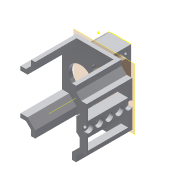
# Autodesk Inventor part: 30_Cube_Z_Focus_MGN_NEMA_base_v3
Saved by Autodesk Inventor 2019.4 (Build 234330000, 330)
## iProperties
Created: 2021-04-25
Part Number: 30_Cube_Z_Focus_MGN_NEMA_base_v3
Material: Generic
Document SubType Name: Modeling
Designer: diederichbenedict
Density: 1 g/cm^3
Appearance: Smooth - White
Author: diederichbenedict
Autodesk Inventor part; units mm, degrees
ref_plane "YZ Plane" through (0, 0, 0) normal (1, 0, 0) x (0, 1, 0)
ref_plane "XZ Plane" through (0, 0, 0) normal (0, 1, 0) x (-1, 0, 0)
ref_plane "XY Plane" through (0, 0, 0) normal (0, 0, 1) x (1, 0, 0)
ref_plane "Work Plane1" through (0, 0, 0) normal (0, 0, 1) x (1, 0, 0)
sketch "Sketch1" plane through (0, 0, 0) normal (0, 0, 1) x (1, 0, 0)
  arc A0 (24.85, 22.85) -> (22.85, 24.85) centre (22.85, 22.85) ccw construction
  line L0 (22.85, 24.85) -> (-16.97, 24.85) construction
  line L1 (-16.97, 24.85) -> (-16.97, 21.15) construction
  line L2 (-16.97, 21.15) -> (16.97, 21.15) construction
  line L3 (16.97, 16.97) -> (16.97, 21.15) construction
  line L4 (21.15, 16.97) -> (16.97, 16.97) construction
  line L5 (21.15, 16.97) -> (21.15, -16.97) construction
  line L6 (21.15, -16.97) -> (24.85, -16.97) construction
  line L7 (24.85, -16.97) -> (24.85, 22.85) construction
  line L8 (23.75, 23.25) -> (23.75, 18.15) construction
  arc A1 (23.25, 17.65) -> (23.75, 18.15) centre (23.25, 18.15) ccw construction
  line L9 (23.25, 17.65) -> (20.8937, 17.65) construction
  arc A2 (20.5239, 17.8134) -> (20.8937, 17.65) centre (20.8937, 18.15) ccw construction
  line L10 (20.5239, 17.8134) -> (17.7803, 20.8273) construction
  arc A3 (17.65, 21.1639) -> (17.7803, 20.8273) centre (18.15, 21.1639) ccw construction
  line L11 (17.65, 21.1639) -> (17.65, 23.25) construction
  arc A4 (18.15, 23.75) -> (17.65, 23.25) centre (18.15, 23.25) ccw construction
  line L12 (18.15, 23.75) -> (23.25, 23.75) construction
  arc A5 (23.75, 23.25) -> (23.25, 23.75) centre (23.25, 23.25) ccw construction
  arc A6 (-24.85, -22.85) -> (-22.85, -24.85) centre (-22.85, -22.85) ccw construction
  line L13 (-22.85, -24.85) -> (16.97, -24.85) construction
  line L14 (16.97, -24.85) -> (16.97, -21.15) construction
  line L15 (16.97, -21.15) -> (-16.97, -21.15) construction
  line L16 (-16.97, -16.97) -> (-16.97, -21.15) construction
  line L17 (-21.15, -16.97) -> (-16.97, -16.97) construction
  line L18 (-21.15, -16.97) -> (-21.15, 16.97) construction
  line L19 (-21.15, 16.97) -> (-24.85, 16.97) construction
  line L20 (-24.85, 16.97) -> (-24.85, -22.85) construction
  line L21 (-20.8273, -17.7803) -> (-17.8134, -20.5239) construction
  arc A7 (-17.65, -20.8937) -> (-17.8134, -20.5239) centre (-18.15, -20.8937) ccw construction
  line L22 (-17.65, -20.8937) -> (-17.65, -23.25) construction
  arc A8 (-18.15, -23.75) -> (-17.65, -23.25) centre (-18.15, -23.25) ccw construction
  line L23 (-18.15, -23.75) -> (-23.25, -23.75) construction
  arc A9 (-23.75, -23.25) -> (-23.25, -23.75) centre (-23.25, -23.25) ccw construction
  line L24 (-23.75, -23.25) -> (-23.75, -18.15) construction
  arc A10 (-23.25, -17.65) -> (-23.75, -18.15) centre (-23.25, -18.15) ccw construction
  line L25 (-23.25, -17.65) -> (-21.1639, -17.65) construction
  arc A11 (-20.8273, -17.7803) -> (-21.1639, -17.65) centre (-21.1639, -18.15) ccw construction
  arc A12 (-22.85, 24.85) -> (-24.85, 22.85) centre (-22.85, 22.85) ccw construction
  line L26 (-22.85, 24.85) -> (16.97, 24.85) construction
  line L27 (16.97, 24.85) -> (16.97, 21.15) construction
  line L28 (16.97, 21.15) -> (-16.97, 21.15) construction
  line L29 (-16.97, 16.97) -> (-16.97, 21.15) construction
  line L30 (-21.15, 16.97) -> (-16.97, 16.97) construction
  line L31 (-21.15, 16.97) -> (-21.15, -16.97) construction
  line L32 (-21.15, -16.97) -> (-24.85, -16.97) construction
  line L33 (-24.85, -16.97) -> (-24.85, 22.85) construction
  line L34 (-20.8273, 17.7803) -> (-17.8134, 20.5239) construction
  arc A13 (-17.8134, 20.5239) -> (-17.65, 20.8937) centre (-18.15, 20.8937) ccw construction
  line L35 (-17.65, 20.8937) -> (-17.65, 23.25) construction
  arc A14 (-17.65, 23.25) -> (-18.15, 23.75) centre (-18.15, 23.25) ccw construction
  line L36 (-18.15, 23.75) -> (-23.25, 23.75) construction
  arc A15 (-23.25, 23.75) -> (-23.75, 23.25) centre (-23.25, 23.25) ccw construction
  line L37 (-23.75, 23.25) -> (-23.75, 18.15) construction
  arc A16 (-23.75, 18.15) -> (-23.25, 17.65) centre (-23.25, 18.15) ccw construction
  line L38 (-23.25, 17.65) -> (-21.1639, 17.65) construction
  arc A17 (-21.1639, 17.65) -> (-20.8273, 17.7803) centre (-21.1639, 18.15) ccw construction
  arc A18 (22.85, -24.85) -> (24.85, -22.85) centre (22.85, -22.85) ccw construction
  line L39 (22.85, -24.85) -> (-16.97, -24.85) construction
  line L40 (-16.97, -24.85) -> (-16.97, -21.15) construction
  line L41 (-16.97, -21.15) -> (16.97, -21.15) construction
  line L42 (16.97, -16.97) -> (16.97, -21.15) construction
  line L43 (21.15, -16.97) -> (16.97, -16.97) construction
  line L44 (21.15, -16.97) -> (21.15, 16.97) construction
  line L45 (21.15, 16.97) -> (24.85, 16.97) construction
  line L46 (24.85, 16.97) -> (24.85, -22.85) construction
  line L47 (23.75, -23.25) -> (23.75, -18.15) construction
  arc A19 (23.75, -18.15) -> (23.25, -17.65) centre (23.25, -18.15) ccw construction
  line L48 (23.25, -17.65) -> (20.8937, -17.65) construction
  arc A20 (20.8937, -17.65) -> (20.5239, -17.8134) centre (20.8937, -18.15) ccw construction
  line L49 (20.5239, -17.8134) -> (17.7803, -20.8273) construction
  arc A21 (17.7803, -20.8273) -> (17.65, -21.1639) centre (18.15, -21.1639) ccw construction
  line L50 (17.65, -21.1639) -> (17.65, -23.25) construction
  arc A22 (17.65, -23.25) -> (18.15, -23.75) centre (18.15, -23.25) ccw construction
  line L51 (18.15, -23.75) -> (23.25, -23.75) construction
  arc A23 (23.25, -23.75) -> (23.75, -23.25) centre (23.25, -23.25) ccw construction
  circle A24 centre (0.47, -10.47) radius 1.1 construction
  circle A25 centre (0.47, 12.53) radius 1.025 construction
  line L52 (24.85, 16.87) -> (16.87, 16.87)
  line L53 (16.87, 16.87) -> (16.87, -16.87)
  line L54 (16.87, -16.87) -> (24.85, -16.87)
  line L55 (24.85, -16.87) -> (24.85, 16.87)
  line L56 (-16.87, 24.85) -> (16.87, 24.85)
  line L57 (16.87, 24.85) -> (16.87, 13.87)
  line L58 (16.87, 13.87) -> (-16.87, 13.87)
  line L59 (-16.87, 13.87) -> (-16.87, 24.85)
  line L60 (-16.87, 16.87) -> (-24.85, 16.87)
  line L61 (-24.85, 16.87) -> (-24.85, -16.87)
  line L62 (-24.85, -16.87) -> (-16.87, -16.87)
  line L63 (-16.87, -16.87) -> (-16.87, 16.87)
  line L64 (-16.87, -24.85) -> (16.87, -24.85)
  line L65 (16.87, -24.85) -> (16.87, -13.87)
  line L66 (16.87, -13.87) -> (-16.87, -13.87)
  line L67 (-16.87, -13.87) -> (-16.87, -24.85)
  arc A26 (12.6573, -5.8482) -> (12.7994, -6.05) centre (12.9383, -5.8013) ccw construction
  line L68 (12.7994, -6.05) -> (16.97, -6.05) construction
  line L69 (16.97, -6.05) -> (16.97, 6.05) construction
  line L70 (12.7994, 6.05) -> (16.97, 6.05) construction
  arc A27 (12.7994, 6.05) -> (12.6573, 5.8482) centre (12.9383, 5.8013) ccw construction
  arc A28 (12.2641, 5.5514) -> (12.6573, 5.8482) centre (11.7553, 6.6343) ccw construction
  arc A29 (12.2641, 5.5514) -> (12.1529, 5.425) centre (12.3846, 5.3332) ccw construction
  line L71 (12.1141, 4.928) -> (12.1529, 5.425) construction
  arc A30 (11.8955, 4.7) -> (12.1141, 4.928) centre (11.8656, 4.9475) ccw construction
  line L72 (11.4444, 4.7) -> (11.8955, 4.7) construction
  arc A31 (11.1961, 4.9275) -> (11.4444, 4.7) centre (11.4444, 4.9493) ccw construction
  line L73 (11.1642, 5.293) -> (11.1961, 4.9275) construction
  arc A32 (11.1642, 5.293) -> (11.0112, 5.5514) centre (10.9164, 5.3208) ccw construction
  arc A33 (10.4933, 5.8954) -> (11.0112, 5.5514) centre (11.4026, 6.7024) ccw construction
  arc A34 (10.4933, 5.8954) -> (10.27, 6.05) centre (10.2627, 5.8008) ccw construction
  line L74 (9.67, 6.05) -> (10.27, 6.05) construction
  line L75 (9.17, 5.55) -> (9.67, 6.05) construction
  line L76 (9.17, 5.55) -> (9.17, -5.55) construction
  line L77 (9.17, -5.55) -> (9.67, -6.05) construction
  line L78 (9.67, -6.05) -> (10.27, -6.05) construction
  arc A35 (10.27, -6.05) -> (10.4933, -5.8954) centre (10.2627, -5.8008) ccw construction
  arc A36 (11.0112, -5.5514) -> (10.4933, -5.8954) centre (11.4026, -6.7024) ccw construction
  arc A37 (11.0112, -5.5514) -> (11.1642, -5.293) centre (10.9164, -5.3208) ccw construction
  line L79 (11.1642, -5.293) -> (11.1961, -4.9275) construction
  arc A38 (11.4444, -4.7) -> (11.1961, -4.9275) centre (11.4444, -4.9493) ccw construction
  line L80 (11.4444, -4.7) -> (11.8955, -4.7) construction
  arc A39 (12.1141, -4.928) -> (11.8955, -4.7) centre (11.8656, -4.9475) ccw construction
  line L81 (12.1141, -4.928) -> (12.1529, -5.425) construction
  arc A40 (12.1529, -5.425) -> (12.2641, -5.5514) centre (12.3846, -5.3332) ccw construction
  arc A41 (12.6573, -5.8482) -> (12.2641, -5.5514) centre (11.7553, -6.6343) ccw construction
  point P0 (0, 0)
extrude "Extrusion1" add sketch "Sketch1" along normal blind 3 contours L55 L54 L53 L52 | L53 L58 L59 L56 L57 | L65 L64 L67 L63 L66 L53 | L63 L62 L61 L60 L59
chamfer "Chamfer1" distance 3.9 angle 45 4 edges at (16.87, -16.87, 1.5) (-16.87, -16.87, 1.5) (-16.87, 16.87, 1.5) (16.87, 16.87, 1.5)
sketch "Sketch2" plane through (0, 0, 3) normal (0, 0, 1) x (1, 0, 0)
  line L0 (-16.87, -13.87) -> (-16.87, 13.87) projected
  line L1 (-16.87, 13.87) -> (16.87, 13.87) projected
  line L2 (16.87, 13.87) -> (16.87, -13.87) projected
  line L3 (16.87, -13.87) -> (-16.87, -13.87) projected
  line L4 (-16.87, -20.77) -> (-16.87, -24.85) projected
  line L5 (-16.87, -24.85) -> (16.87, -24.85) projected
  line L6 (16.87, -24.85) -> (16.87, -20.77) projected
  line L7 (20.77, -16.87) -> (16.87, -20.77) projected
  line L8 (20.77, -16.87) -> (24.85, -16.87) projected
  line L9 (24.85, -16.87) -> (24.85, 16.87) projected
  line L10 (24.85, 16.87) -> (20.77, 16.87) projected
  line L11 (16.87, 20.77) -> (20.77, 16.87) projected
  line L12 (16.87, 20.77) -> (16.87, 24.85) projected
  line L13 (16.87, 24.85) -> (-16.87, 24.85) projected
  line L14 (-16.87, 24.85) -> (-16.87, 20.77) projected
  line L15 (-20.77, 16.87) -> (-16.87, 20.77) projected
  line L16 (-20.77, 16.87) -> (-24.85, 16.87) projected
  line L17 (-24.85, 16.87) -> (-24.85, -16.87) projected
  line L18 (-24.85, -16.87) -> (-20.77, -16.87) projected
  line L19 (-16.87, -20.77) -> (-20.77, -16.87) projected
  line L20 (13.8689, -19.5269) -> (13.8689, -21.8489)
  line L21 (-13.8689, -21.8489) -> (-13.8689, -19.5269)
  line L22 (-13.8689, -19.5269) -> (-19.5269, -13.8689)
  line L23 (-19.5269, -13.8689) -> (-21.8489, -13.8689)
  line L24 (-21.8489, 13.8689) -> (-19.5269, 13.8689)
  line L25 (-19.5269, 13.8689) -> (-13.8689, 19.5269)
  line L26 (-13.8689, 19.5269) -> (-13.8689, 21.8489)
  line L27 (13.8689, 21.8489) -> (13.8689, 19.5269)
  line L28 (13.8689, 19.5269) -> (19.5269, 13.8689)
  line L29 (19.5269, 13.8689) -> (21.8489, 13.8689)
  line L30 (21.8489, -13.8689) -> (19.5269, -13.8689)
  line L31 (19.5269, -13.8689) -> (13.8689, -19.5269)
  line L32 (13.8689, -21.8489) -> (13.8689, -24.85)
  line L33 (16.87, -24.85) -> (-16.87, -24.85) projected
  line L34 (21.8489, -13.8689) -> (24.85, -13.8689)
  line L35 (24.85, -16.87) -> (24.85, 16.87) projected
  line L36 (21.8489, 13.8689) -> (24.85, 13.8689)
  line L37 (13.8689, 21.8489) -> (13.8689, 24.85)
  line L38 (-13.8689, 21.8489) -> (-13.8689, 24.85)
  line L39 (-21.8489, 13.8689) -> (-24.85, 13.8689)
  line L40 (-21.8489, -13.8689) -> (-24.85, -13.8689)
  line L41 (-13.8689, -21.8489) -> (-13.8689, -24.85)
  line L42 (13.8689, -21.8489) -> (11.5469, -21.8489)
  line L43 (-11.5469, -21.8489) -> (-13.8689, -21.8489)
  line L44 (21.8489, 13.8689) -> (21.8489, 11.5469)
  line L45 (21.8489, -11.5469) -> (21.8489, -13.8689)
  line L46 (-21.8489, -13.8689) -> (-21.8489, -11.5469)
  line L47 (-21.8489, 11.5469) -> (-21.8489, 13.8689)
  line L48 (-13.8689, 21.8489) -> (-11.5469, 21.8489)
  line L49 (11.5469, 21.8489) -> (13.8689, 21.8489)
  point P0 (0, 0)
  dimension "d13" = 3.0011
  constraints: 56 end point, 20 point on line, 3 perpendicular, 1 parallel, 7 other
  measures "d13" distance between parallel lines of L6 L20
ref_plane "Work Plane2" through (-16.97, -24.85, 34.1) normal (0, 0, -1) x (0, 1, 0)
extrude "Extrusion2" add sketch "Sketch2" along normal up to surface (31.1 mm away) contours L32 L20 L31 L30 L34 L9 L8 L7 L6 L5
pattern_circular "Circular Pattern1" count 4 over 360 about axis through (0, 0, 17.13) along (0, 0, -1) of "Extrusion2"
sketch "Sketch3" plane through (-24.85, -13.8689, 34.1) normal (0, 0, 1) x (1, 0, 0)
  circle A0 centre (13.82, 14.8989) radius 1.5 projected
  line L0 (10.9811, -5.658) -> (5.3231, 0) projected
  line L1 (5.3231, 0) -> (0, 0) projected
  line L2 (0, 0) -> (0, -3.0011) projected
  line L3 (0, -3.0011) -> (4.08, -3.0011) projected
  line L4 (4.08, -3.0011) -> (7.98, -6.9011) projected
  line L5 (7.98, -6.9011) -> (7.98, -10.9811) projected
  line L6 (7.98, -10.9811) -> (10.9811, -10.9811) projected
  line L7 (10.9811, -10.9811) -> (10.9811, -5.658) projected
  line L8 (5.3231, 27.7378) -> (10.9811, 33.3958) projected
  line L9 (10.9811, 33.3958) -> (10.9811, 38.7189) projected
  line L10 (10.9811, 38.7189) -> (7.98, 38.7189) projected
  line L11 (7.98, 38.7189) -> (7.98, 34.6389) projected
  line L12 (7.98, 34.6389) -> (4.08, 30.7389) projected
  line L13 (4.08, 30.7389) -> (0, 30.7389) projected
  line L14 (0, 30.7389) -> (0, 27.7378) projected
  line L15 (0, 27.7378) -> (5.3231, 27.7378) projected
  line L16 (10.9811, -10.9811) -> (16.9811, -10.9811)
  line L17 (16.9811, 38.7189) -> (10.9811, 38.7189)
  line L18 (0, 0) -> (0, 27.7378)
  line L19 (0, 0) -> (5.3231, 0)
  line L20 (5.3231, 0) -> (5.3231, 27.7378)
  line L21 (5.3231, 27.7378) -> (0, 27.7378)
  line L22 (0, 27.7378) -> (0, 0)
  line L23 (5.3231, 0) -> (0, 0) projected
  line L24 (5.3231, 0) -> (10.9811, -5.658)
  line L25 (10.9811, 33.3958) -> (5.3231, 27.7378)
  line L26 (38.7189, 38.7189) -> (38.7189, 33.3958) projected
  line L27 (38.7189, -5.658) -> (38.7189, -10.9811) projected
  line L28 (10.9811, -10.9811) -> (38.7189, -10.9811)
  line L29 (38.7189, -10.9811) -> (38.7189, -5.658)
  line L30 (38.7189, -5.658) -> (10.9811, -5.658)
  line L31 (10.9811, -5.658) -> (10.9811, -10.9811)
  line L32 (10.9811, 38.7189) -> (10.9811, 33.3958) projected
  line L33 (10.9811, 38.7189) -> (38.7189, 38.7189)
  line L34 (38.7189, 38.7189) -> (38.7189, 33.3958)
  line L35 (38.7189, 33.3958) -> (10.9811, 33.3958)
  line L36 (10.9811, 33.3958) -> (10.9811, 38.7189)
  line L37 (16.9811, -10.9811) -> (16.9811, -5.658)
  line L38 (16.9811, 33.3958) -> (16.9811, 38.7189)
  line L39 (10.9811, 38.7189) -> (10.9811, 33.3958)
  line L40 (10.9811, -5.658) -> (10.9811, -10.9811)
  line L41 (10.9811, -5.658) -> (10.9811, 0)
  line L42 (10.9811, 27.7378) -> (10.9811, 33.3958)
  line L43 (49.7, 0) -> (44.3769, 0) projected
  line L44 (44.3769, 27.7378) -> (49.7, 27.7378) projected
  line L45 (44.3769, 27.7378) -> (49.7, 27.7378)
  line L46 (49.7, 27.7378) -> (49.7, 0)
  line L47 (49.7, 0) -> (44.3769, 0)
  line L48 (44.3769, 0) -> (44.3769, 27.7378)
  point P0 (24.85, 13.8689)
  dimension "d19" = 6
  constraints: 54 end point, 14 equal length, 6 perpendicular, 5 horizontal, 4 point on line, 3 vertical
  measures "d19" distance of L17.end L17.start
extrude "Extrusion3" add sketch "Sketch3" against normal blind 1 contours L7 L6 L5 L4 L3 L2 L1 L0 | L15 L14 L13 L12 L11 L10 L9 L8 | L43 L48 L44 L46
sketch "Sketch4" plane through (24.85, -16.87, 0) normal (1, 0, 0) x (0, 0, -1)
  line L0 (37.9, 11.3739) -> (37.9, 18.453) construction
  line L1 (23.6194, 18.453) -> (37.9, 18.453) construction
  arc A0 (22.1806, 18.453) -> (23.6194, 18.453) centre (22.9, 16.8577) ccw construction
  line L2 (-1.3806, 18.453) -> (22.1806, 18.453) construction
  arc A1 (-2.8194, 18.453) -> (-1.3806, 18.453) centre (-2.1, 16.8577) ccw construction
  line L3 (-31.3806, 18.453) -> (-2.8194, 18.453) construction
  arc A2 (-32.8194, 18.453) -> (-31.3806, 18.453) centre (-32.1, 16.8577) ccw construction
  line L4 (-42.1, 18.453) -> (-32.8194, 18.453) construction
  line L5 (-42.1, 11.3739) -> (-42.1, 18.453) construction
  line L6 (-42.1, 11.3739) -> (37.9, 11.3739) construction
  line L7 (37.9, 19.2506) -> (37.9, 22.3415) construction
  line L8 (-42.1, 22.3415) -> (37.9, 22.3415) construction
  line L9 (-42.1, 19.2506) -> (-42.1, 22.3415) construction
  line L10 (-42.1, 19.2506) -> (37.9, 19.2506) construction
  line L11 (-3, 3.0011) -> (-3, 30.7389) construction
  line L12 (-34.1, 33.84) -> (-34.1, -5.98) construction
  line L13 (-3, 11.3739) -> (-34.1, 11.3739)
  line L14 (-34.1, 11.3739) -> (-34.1, 22.3415)
  line L15 (-34.1, 22.3415) -> (-3, 22.3415)
  line L16 (-3, 22.3415) -> (-3, 11.3739)
  line L17 (-34.1, 11.3739) -> (-32.1, 11.3739)
  line L18 (-32.1, 11.3739) -> (-32.1, 3.0011)
  line L19 (-32.1, 3.0011) -> (-34.1, 3.0011)
  line L20 (-34.1, 3.0011) -> (-34.1, 11.3739)
  line L21 (-34.1, 22.3415) -> (-32.1, 22.3415)
  line L22 (-32.1, 22.3415) -> (-32.1, 30.7389)
  line L23 (-32.1, 30.7389) -> (-34.1, 30.7389)
  line L24 (-34.1, 30.7389) -> (-34.1, 22.3415)
  point P0 (0, 16.87)
  dimension "d24" = 2
  constraints: 24 end point, 6 parallel, 5 point on line, 3 horizontal, 3 perpendicular
  measures "d24" distance of L18.end L19.end
ref_plane "Work Plane3" through (16.97, -5.4961, -37.9) normal (1, 0, 0) x (0, 1, 0)
extrude "Extrusion4" add sketch "Sketch4" against normal up to surface (7.88 mm away) contours L13 L14 L15 L16
sketch "Sketch5" plane through (24.85, -16.87, 0) normal (1, 0, 0) x (0, 0, -1)
  circle A0 centre (-32.1, 16.87) radius 1.4
  circle A1 centre (-2.1, 16.87) radius 1.4
  line L0 (0, -7.98) -> (-34.1, -7.98) projected
  line L1 (0, 41.72) -> (-34.1, 41.72) projected
  line L2 (0, -7.98) -> (-34.1, -7.98) projected
  point P0 (0, 16.87)
  dimension "d25" = 2.8
  dimension "d26" = 2.8
  dimension "d86" = 49.7
  dimension "d87" = 24.85
  dimension "d88" = 0
  constraints: 2 centre point
  measures "d25" diameter of A0
  measures "d26" diameter of A1
  measures "d86" distance between parallel lines of L1 L2
  measures "d87" distance from line of A0.centre L1
  measures "d88" vertical distance of A1.centre A0.centre
extrude "Extrusion5" cut sketch "Sketch5" against normal blind 10
pattern_linear "Rectangular Pattern1" count 4 spacing 7.5 along (0, 0, 1) of "Extrusion5"
sketch "Sketch7" plane through (0, 0, 0) normal (0, 0, -1) x (-1, 0, 0)
  arc A0 (18.93, 12.43) -> (22.43, 8.93) centre (22.43, 12.43) ccw construction
  line L0 (18.93, 12.43) -> (18.93, 14.53) construction
  line L1 (3.13, 14.53) -> (18.93, 14.53) construction
  line L2 (3.13, 14.53) -> (3.13, 12.43) construction
  arc A1 (-0.37, 8.93) -> (3.13, 12.43) centre (-0.37, 12.43) ccw construction
  line L3 (-0.37, 8.93) -> (-2.47, 8.93) construction
  line L4 (-2.47, -6.87) -> (-2.47, 8.93) construction
  line L5 (-2.47, -6.87) -> (-0.37, -6.87) construction
  arc A2 (3.13, -10.37) -> (-0.37, -6.87) centre (-0.37, -10.37) ccw construction
  line L6 (3.13, -10.37) -> (3.13, -12.47) construction
  line L7 (18.93, -12.47) -> (3.13, -12.47) construction
  line L8 (18.93, -12.47) -> (18.93, -10.37) construction
  arc A3 (22.43, -6.87) -> (18.93, -10.37) centre (22.43, -10.37) ccw construction
  line L9 (22.43, -6.87) -> (24.53, -6.87) construction
  line L10 (24.53, 8.93) -> (24.53, -6.87) construction
  line L11 (24.53, 8.93) -> (22.43, 8.93) construction
  circle A4 centre (11.03, 1.03) radius 2.5 construction
  arc A5 (-1.5344, 11.2045) -> (0.934, 13.4886) centre (-0.47, 12.53) ccw construction
  circle A6 centre (-0.47, -10.47) radius 1.1 construction
  arc A7 (0.5944, 13.8555) -> (-1.874, 11.5714) centre (-0.47, 12.53) ccw construction
  line L12 (-19.5269, -13.8689) -> (-24.85, -13.8689) construction
  line L13 (-16.87, -1.0724) -> (-16.87, -13.87) construction
  line L14 (-16.87, -13.87) -> (16.87, -13.87) construction
  line L15 (16.87, -13.87) -> (16.87, 13.87) construction
  line L16 (16.87, 13.87) -> (-16.87, 13.87) construction
  line L17 (-19.5269, 13.8689) -> (-13.8689, 19.5269) construction
  line L18 (-13.8689, 19.5269) -> (-13.8689, 24.85) construction
  line L19 (-13.8689, 24.85) -> (13.8689, 24.85) construction
  line L20 (13.8689, 24.85) -> (13.8689, 19.5269) construction
  line L21 (13.8689, 19.5269) -> (19.5269, 13.8689) construction
  line L22 (19.5269, 13.8689) -> (24.85, 13.8689) construction
  line L23 (24.85, 13.8689) -> (24.85, -13.8689) construction
  line L24 (24.85, -13.8689) -> (19.5269, -13.8689) construction
  line L25 (19.5269, -13.8689) -> (13.8689, -19.5269) construction
  line L26 (13.8689, -19.5269) -> (13.8689, -24.85) construction
  line L27 (13.8689, -24.85) -> (-13.8689, -24.85) construction
  line L28 (-13.8689, -24.85) -> (-13.8689, -19.5269) construction
  line L29 (-13.8689, -19.5269) -> (-19.5269, -13.8689) construction
  line L30 (16.87, 13.87) -> (-16.87, 13.87) construction
  line L31 (16.87, 13.87) -> (-19.5258, 13.87) projected
  line L32 (-2.13, 13.87) -> (16.87, 13.87)
  line L33 (16.87, 13.87) -> (16.87, -16.45)
  line L34 (16.87, -16.45) -> (-2.13, -16.45)
  line L35 (-2.13, -16.45) -> (-2.13, 13.87)
  line L36 (16.97, 16.97) -> (-16.97, 16.97)
  line L37 (16.87, 13.87) -> (-2.13, 13.87)
  line L38 (-2.13, 13.87) -> (-2.13, 16.45)
  line L39 (-2.13, 16.45) -> (16.87, 16.45)
  line L40 (16.87, 16.45) -> (16.87, 13.87)
  line L41 (-16.97, -16.97) -> (16.97, -16.97) construction
  line L42 (-16.87, 1.0724) -> (-16.97, 1.0724) projected
  line L43 (-16.97, 1.0724) -> (-16.97, 5.4715) projected
  line L44 (-16.97, 5.4715) -> (-24.85, 5.4715) projected
  line L45 (-24.85, 5.4715) -> (-24.85, 13.8689) projected
  line L46 (-24.85, 13.8689) -> (-19.5269, 13.8689) projected
  line L47 (-24.85, -13.8689) -> (-24.85, -5.4961) projected
  line L48 (-24.85, -5.4961) -> (-16.97, -5.4961) projected
  line L49 (-16.97, -5.4961) -> (-16.97, -1.0724) projected
  line L50 (-16.97, -1.0724) -> (-16.87, -1.0724) projected
  line L51 (-16.87, 13.87) -> (-16.87, 1.0724) projected
  point P0 (0, 0)
  dimension "d35" = 19
  dimension "d36" = 0
  dimension "d74" = 16.45
  dimension "d75" = 16.45
  constraints: 18 end point, 4 parallel, 3 horizontal, 2 perpendicular, 1 point on line, 2 other
  measures "d35" distance between parallel lines of L33 L35
  measures "d36" distance between parallel lines of L33 L15
  measures "d74" distance from line of L39 point (0, 0)
  measures "d75" distance from line of L34 point (0, 0)
ref_plane "Work Plane4" through (-25.03, -12.97, -12) normal (0, 0, 1) x (1, 0, 0)
extrude "Extrusion7" add sketch "Sketch7" along normal blind 22 and the other way blind 3 contours L33 L34 L35 L31 | L31 L38 L39 L40
sketch "Sketch8" plane through (0, 0, 3) normal (0, 0, 1) x (1, 0, 0)
  circle A0 centre (0.47, 12.53) radius 1.025 projected
  arc A1 (8.8, 18.96) -> (8.8, 22.36) centre (8.8, 20.66) ccw projected
  circle A2 centre (0.47, -10.47) radius 1.025 projected
  circle A3 centre (0.47, 11.5) radius 1.0261
  circle A4 centre (0.47, -11.5) radius 1.0306
  point P0 (0, 0)
  dimension "d76" = 12.53
  dimension "d77" = 23
  dimension "d78" = 11.5
  dimension "d79" = 11.5
  constraints: 2 centre point
  measures "d76" vertical distance of point (0, 0) A0.centre
  measures "d77" distance of A2.centre A0.centre
  measures "d78" vertical distance of point (0, 0) A3.centre
  measures "d79" vertical distance of A4.centre point (0, 0)
hole "Hole1" at (0.47, 11.5, 3) at (0.47, -11.5, 3) direction (0, 0, -1) diameter 2.5 end through all counterbore diameter 6 counterbore depth 22
sketch "Sketch9" plane through (2.13, -16.47, -22) normal (0, 0, -1) x (-1, 0, 0)
  circle A0 centre (13.16, 17.5) radius 11 projected
  circle A1 centre (13.16, 17.5) radius 13
  circle A2 centre (13.16, 16.47) radius 12.7687
  circle A3 centre (1.66, 27.97) radius 1.25 projected
  point P0 (2.13, 16.47)
  dimension "d46" = 2
  dimension "d80" = 11.5
  constraints: 2 centre point
  measures "d46" radial gap between concentric circles of A0 A1
  measures "d80" horizontal distance of A2.centre A3.centre
extrude "Extrusion8" cut sketch "Sketch9" against normal blind 3 contours A0 | A2 A1 | A1 A2 picked at (13.602, 5.2544) picked at (13.16, 4.2947)
sketch "Sketch10" plane through (2.13, -16.47, -19) normal (0, 0, -1) x (-1, 0, 0)
  arc A0 (19, 27.8249) -> (19, 5.1151) centre (13.16, 16.47) ccw projected
  circle A1 centre (13.16, 16.47) radius 9
  dimension "d81" = 18
  constraints: 1 centre point, 1 coincident
  measures "d81" diameter of A1
extrude "Extrusion9" cut sketch "Sketch10" against normal up to next
sketch "Sketch12" plane through (24.85, -16.87, 0) normal (1, 0, 0) x (0, 0, -1)
  ellipse E0 centre (-17.053, 16.87) end of major axis (-32.053, 16.87) minor radius 10.6066 projected
  circle A0 centre (-32.1, 16.87) radius 1.4 projected
  circle A1 centre (-24.6, 16.87) radius 1.4 projected
  circle A2 centre (-17.1, 16.87) radius 1.4 projected
  circle A3 centre (-9.6, 16.87) radius 1.4 projected
  circle A4 centre (-2.1, 16.87) radius 1.4 projected
  point P0 (0, 16.87)
  constraints: 1 other
hole "Hole2" at (24.85, 0, 32.1) at (24.85, 0, 24.6) at (24.85, 0, 17.053) at (24.85, 0, 9.6) at (24.85, 0, 2.1) direction (-1, 0, 0) diameter 2.8 depth 8 tip angle 118 counterbore diameter 6 counterbore depth 3
chamfer "Chamfer2" distance 2 angle 45 2 edges at (19.5269, 5.4715, 33.6) (19.5269, -5.4961, 33.6)
fillet "Fillet1" radius 4 2 edges at (-16.87, -16.45, -11) (-16.87, 16.45, -11)
sketch "Sketch14" plane through (0, 0, -22) normal (0, 0, -1) x (-1, 0, 0)
  arc A0 (16.87, 12.45) -> (12.87, 16.45) centre (12.87, 12.45) ccw projected
  line L0 (12.87, 16.45) -> (-2.13, 16.45) projected
  line L1 (-2.13, 16.45) -> (-2.13, -16.45) projected
  line L2 (-2.13, -16.45) -> (12.87, -16.45) projected
  arc A1 (12.87, -16.45) -> (16.87, -12.45) centre (12.87, -12.45) ccw projected
  line L3 (16.87, -12.45) -> (16.87, -11.3549) projected
  arc A2 (16.87, 11.3549) -> (16.87, -11.3549) centre (11.03, 0) ccw projected
  line L4 (16.87, 11.3549) -> (16.87, 12.45) projected
  circle A3 centre (-0.47, 11.5) radius 1.25 projected
  circle A4 centre (-0.47, -11.5) radius 1.25 projected
  arc A5 (22.43, -7.9) -> (18.93, -11.4) centre (22.43, -11.4) ccw construction
  line L5 (22.43, -7.9) -> (24.53, -7.9) construction
  line L6 (24.53, 7.9) -> (24.53, -7.9) construction
  line L7 (24.53, 7.9) -> (22.43, 7.9) construction
  arc A6 (18.93, 11.4) -> (22.43, 7.9) centre (22.43, 11.4) ccw construction
  line L8 (18.93, 11.4) -> (18.93, 13.5) construction
  line L9 (3.13, 13.5) -> (18.93, 13.5) construction
  line L10 (3.13, 13.5) -> (3.13, 11.4) construction
  arc A7 (-0.37, 7.9) -> (3.13, 11.4) centre (-0.37, 11.4) ccw construction
  line L11 (-0.37, 7.9) -> (-2.47, 7.9) construction
  line L12 (-2.47, -7.9) -> (-2.47, 7.9) construction
  line L13 (-2.47, -7.9) -> (-0.37, -7.9) construction
  arc A8 (3.13, -11.4) -> (-0.37, -7.9) centre (-0.37, -11.4) ccw construction
  line L14 (3.13, -11.4) -> (3.13, -13.5) construction
  line L15 (18.93, -13.5) -> (3.13, -13.5) construction
  line L16 (18.93, -13.5) -> (18.93, -11.4) construction
  circle A9 centre (11.03, 0) radius 2.5 construction
  circle A10 centre (22.53, 11.5) radius 1 construction
  point P0 (0, 0)
sketch "Sketch15" plane through (0, 0, 3) normal (0, 0, 1) x (1, 0, 0)
  arc A0 (12.6573, -5.7482) -> (12.7994, -5.95) centre (12.9383, -5.7012) ccw projected
  line L0 (12.7994, -5.95) -> (16.97, -5.95) projected
  line L1 (16.97, -5.95) -> (16.97, 6.15) projected
  line L2 (12.7994, 6.15) -> (16.97, 6.15) projected
  arc A1 (12.7994, 6.15) -> (12.6573, 5.9482) centre (12.9383, 5.9013) ccw projected
  arc A2 (12.2641, 5.6514) -> (12.6573, 5.9482) centre (11.7553, 6.7343) ccw projected
  arc A3 (12.2641, 5.6514) -> (12.1529, 5.525) centre (12.3846, 5.4332) ccw projected
  line L3 (12.1141, 5.028) -> (12.1529, 5.525) projected
  arc A4 (11.8955, 4.8) -> (12.1141, 5.028) centre (11.8656, 5.0475) ccw projected
  line L4 (11.4444, 4.8) -> (11.8955, 4.8) projected
  arc A5 (11.1961, 5.0276) -> (11.4444, 4.8) centre (11.4444, 5.0493) ccw projected
  line L5 (11.1642, 5.393) -> (11.1961, 5.0276) projected
  arc A6 (11.1642, 5.393) -> (11.0112, 5.6514) centre (10.9164, 5.4208) ccw projected
  arc A7 (10.4933, 5.9954) -> (11.0112, 5.6514) centre (11.4026, 6.8024) ccw projected
  arc A8 (10.4933, 5.9954) -> (10.27, 6.15) centre (10.2627, 5.9009) ccw projected
  line L6 (9.67, 6.15) -> (10.27, 6.15) projected
  line L7 (9.17, 5.65) -> (9.67, 6.15) projected
  line L8 (9.17, 5.65) -> (9.17, -5.45) projected
  line L9 (9.17, -5.45) -> (9.67, -5.95) projected
  line L10 (9.67, -5.95) -> (10.27, -5.95) projected
  arc A9 (10.27, -5.95) -> (10.4933, -5.7954) centre (10.2627, -5.7008) ccw projected
  arc A10 (11.0112, -5.4514) -> (10.4933, -5.7954) centre (11.4026, -6.6024) ccw projected
  arc A11 (11.0112, -5.4514) -> (11.1642, -5.193) centre (10.9164, -5.2208) ccw projected
  line L11 (11.1642, -5.193) -> (11.1961, -4.8275) projected
  arc A12 (11.4444, -4.6) -> (11.1961, -4.8275) centre (11.4444, -4.8493) ccw projected
  line L12 (11.4444, -4.6) -> (11.8955, -4.6) projected
  arc A13 (12.1141, -4.828) -> (11.8955, -4.6) centre (11.8656, -4.8474) ccw projected
  line L13 (12.1141, -4.828) -> (12.1529, -5.325) projected
  arc A14 (12.1529, -5.325) -> (12.2641, -5.4514) centre (12.3846, -5.2332) ccw projected
  arc A15 (12.6573, -5.7482) -> (12.2641, -5.4514) centre (11.7553, -6.5343) ccw projected
  circle A16 centre (-11.03, 0) radius 9 projected
  arc A17 (2.3093, 13.87) -> (2.13, 9.0011) centre (0.47, 11.5) ccw projected
  line L14 (2.3093, 13.87) -> (16.87, 13.87) projected
  line L15 (16.87, 13.87) -> (16.87, 1.0724) projected
  line L16 (16.87, 1.0724) -> (16.97, 1.0724) projected
  line L17 (16.97, 1.0724) -> (16.97, 5.4715) projected
  line L18 (16.97, 5.4715) -> (24.85, 5.4715) projected
  line L19 (24.85, 5.4715) -> (24.85, 13.8689) projected
  line L20 (24.85, 13.8689) -> (19.5269, 13.8689) projected
  line L21 (19.5269, 13.8689) -> (13.8689, 19.5269) projected
  line L22 (13.8689, 19.5269) -> (13.8689, 24.85) projected
  line L23 (13.8689, 24.85) -> (-13.8689, 24.85) projected
  line L24 (-13.8689, 24.85) -> (-13.8689, 19.5269) projected
  line L25 (-13.8689, 19.5269) -> (-19.5269, 13.8689) projected
  line L26 (-19.5269, 13.8689) -> (-24.85, 13.8689) projected
  line L27 (-24.85, 13.8689) -> (-24.85, -13.8689) projected
  line L28 (-24.85, -13.8689) -> (-19.5269, -13.8689) projected
  line L29 (-19.5269, -13.8689) -> (-13.8689, -19.5269) projected
  line L30 (-13.8689, -19.5269) -> (-13.8689, -24.85) projected
  line L31 (-13.8689, -24.85) -> (13.8689, -24.85) projected
  line L32 (13.8689, -24.85) -> (13.8689, -19.5269) projected
  line L33 (13.8689, -19.5269) -> (19.5269, -13.8689) projected
  line L34 (19.5269, -13.8689) -> (24.85, -13.8689) projected
  line L35 (24.85, -13.8689) -> (24.85, -5.4961) projected
  line L36 (24.85, -5.4961) -> (16.97, -5.4961) projected
  line L37 (16.97, -5.4961) -> (16.97, -1.0724) projected
  line L38 (16.97, -1.0724) -> (16.87, -1.0724) projected
  line L39 (16.87, -1.0724) -> (16.87, -13.87) projected
  line L40 (16.87, -13.87) -> (2.3093, -13.87) projected
  arc A18 (2.13, -9.0011) -> (2.3093, -13.87) centre (0.47, -11.5) ccw projected
  line L41 (2.13, -9.0011) -> (2.13, 9.0011) projected
  line L42 (2.3093, 13.87) -> (16.87, 13.87) projected
  line L43 (16.87, 13.87) -> (14.37, 13.87)
  line L44 (14.37, 13.87) -> (14.37, 6.15)
  line L45 (14.37, 6.15) -> (16.87, 6.15)
  line L46 (16.87, 6.15) -> (16.87, 13.87)
  line L47 (16.87, -1.0724) -> (16.87, -13.87) projected
  line L48 (16.87, -13.87) -> (14.37, -13.87)
  line L49 (14.37, -13.87) -> (14.37, -5.95)
  line L50 (14.37, -5.95) -> (16.87, -5.95)
  line L51 (16.87, -5.95) -> (16.87, -13.87)
  point P0 (0, 0)
  dimension "d82" = 2.5
  dimension "d83" = 7.72
  constraints: 16 end point, 4 parallel, 3 point on line, 2 horizontal, 2 perpendicular
  measures "d82" distance of L45.end L44.end
  measures "d83" distance of L44.end L43.end
ref_plane "Work Plane5" through (-16.97, -16.97, 0) normal (0, 0, 1) x (1, 0, 0)
extrude "Extrusion12" add sketch "Sketch15" against normal up to surface (3 mm away) contours L0 L39 L40 L49 | L2 L44 L14 L15
equation "\"d2\" = d1"
equation "\"d3\" = d1"
equation "\"d4\" = d1"
equation "\"d5\" = d1"
equation "\"d1\" = 0.1"
body "Solid1"
